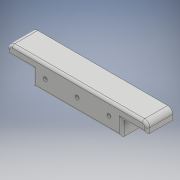
# Autodesk Inventor part: foot_front
Saved by Autodesk Inventor 2018 (Build 220112000, 112)
## iProperties
Created: 2018-05-29
Part Number: foot_front
Material: Generic
Document SubType Name: Modeling
Designer: bitbots
Density: 1 g/cm^3
Appearance: Default
Author: bitbots
Autodesk Inventor part; units mm, degrees
ref_plane "YZ Plane" through (0, 0, 0) normal (1, 0, 0) x (0, 1, 0)
ref_plane "XZ Plane" through (0, 0, 0) normal (0, 1, 0) x (-1, 0, 0)
sketch "Sketch1" plane through (0, 0, 0) normal (0, 1, 0) x (-1, 0, 0)
  line L0 (-35, 10) -> (35, 10)
  line L1 (35, 10) -> (35, -10)
  line L2 (35, -10) -> (-35, -10)
  line L3 (-35, -10) -> (-35, 10)
  line L4 (-35, 10) -> (35, -10) construction
  line L5 (35, 10) -> (-35, -10) construction
  line L6 (0, 0) -> (25, 0)
  line L7 (0, 0) -> (-25, 0)
  circle A0 centre (25, 0) radius 1.5
  circle A1 centre (-25, 0) radius 1.5
  circle A2 centre (0, 0) radius 1.5
  dimension "d0" = 70
  dimension "d1" = 20
  dimension "d2" = 25
  dimension "d3" = 25
  dimension "d4" = 3
  dimension "d5" = 3
  dimension "d8" = 3
  constraints: 16 end point, 3 centre point, 3 coincident, 3 parallel, 2 horizontal, 2 midpoint, 1 perpendicular
  measures "d0" distance of L1.end L2.end
  measures "d1" distance of L0.end L1.end
  measures "d2" distance of L6.start L6.end
  measures "d3" distance of L6.start L7.end
  measures "d4" diameter of A0
  measures "d5" diameter of A1
  measures "d8" diameter of A2
extrude "Extrusion1" add sketch "Sketch1" along normal blind 20
sketch "Sketch2" plane through (0, 20, 0) normal (0, 1, 0) x (1, 0, 0)
  circle A0 centre (0, 0) radius 1.5 projected
  circle A1 centre (25, 0) radius 1.5 projected
  circle A2 centre (-25, 0) radius 1.5 projected
  line L0 (-35, -10) -> (35, -10) projected
  line L1 (35, -10) -> (35, 10) projected
  line L2 (35, 10) -> (-35, 10) projected
  line L3 (-35, 10) -> (-35, -10) projected
  line L4 (-35, 10) -> (-35, -10) projected
  line L5 (-35, -10) -> (-55, -10)
  line L6 (-55, -10) -> (-55, -2)
  line L7 (-55, -2) -> (-35, -2)
  line L8 (-35, -2) -> (-35, -10)
  line L9 (35, -10) -> (55, -10)
  line L10 (55, -10) -> (55, -2)
  line L11 (55, -2) -> (35, -2)
  line L12 (35, -2) -> (35, -10)
  dimension "d9" = 20
  dimension "d10" = 8
  dimension "d11" = 20
  dimension "d12" = 8
  constraints: 16 end point, 4 parallel, 2 horizontal, 2 perpendicular
  measures "d9" distance of L6.end L7.end
  measures "d10" distance of L5.end L6.end
  measures "d11" distance of L11.end L10.end
  measures "d12" distance of L10.end L9.end
extrude "Extrusion2" add sketch "Sketch2" against normal up to surface (20 mm away) contours L5 L6 L7 L3 | L1 L11 L10 L9
ref_plane "Work Plane1" through (0, 16, 0) normal (0, 1, 0) x (1, 0, 0)
sketch "Sketch3" plane through (0, 16, 0) normal (0, 1, 0) x (1, 0, 0)
  circle A0 centre (0, 0) radius 1.5 construction
  circle A1 centre (25, 0) radius 1.5 construction
  circle A2 centre (-25, 0) radius 1.5 construction
  line L0 (-55, -10) -> (55, -10) construction
  line L1 (55, -10) -> (55, -2) construction
  line L2 (55, -2) -> (35, -2) construction
  line L3 (35, -2) -> (35, 10) construction
  line L4 (35, 10) -> (-35, 10) construction
  line L5 (-35, 10) -> (-35, -2) construction
  line L6 (-35, -2) -> (-55, -2) construction
  line L7 (-55, -2) -> (-55, -10) construction
  circle A3 centre (-25, 0) radius 1.5 construction
  line L8 (-25, 0) -> (-27.6, 0) construction
  line L9 (-27.6, 1.5011) -> (-25, 3.0022)
  line L10 (-25, 3.0022) -> (-22.4, 1.5011)
  line L11 (-22.4, 1.5011) -> (-22.4, -1.5011)
  line L12 (-22.4, -1.5011) -> (-25, -3.0022)
  line L13 (-25, -3.0022) -> (-27.6, -1.5011)
  line L14 (-27.6, -1.5011) -> (-27.6, 1.5011)
  line L15 (-35, 10) -> (35, 10) projected
  line L16 (-27.6, 1.5011) -> (-22.4, 1.5011)
  line L17 (-22.4, 1.5011) -> (-22.4, 10)
  line L18 (-22.4, 10) -> (-27.6, 10)
  line L19 (-27.6, 10) -> (-27.6, 1.5011)
  dimension "d17" = 2.6
  constraints: 22 end point, 2 horizontal, 2 parallel, 1 coincident, 1 midpoint, 1 perpendicular, 1 point on line, 13 other
  measures "d17" distance of L8.start L8.end
extrude "Extrusion3" cut sketch "Sketch3" against normal blind 3
pattern_linear "Rectangular Pattern1" count 3 spacing 25 along (1, 0, 0) of "Extrusion3"
fillet "Fillet1" radius 2 8 edges at (0, 0, 10) (0, 0, -10) (-35, 0, -4) (-45, 0, 2) (-55, 0, 6) (35, 0, -4) (45, 0, 2) (55, 0, 6)
fillet "Fillet1" radius 4 2 edges at (55, 10, 10) (-55, 10, 10)
body "Solid1"
